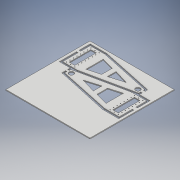
# Autodesk Inventor part: W1support
Saved by Autodesk Inventor 2017 (Build 210142000, 142)
## iProperties
Created: 2016-10-09
Part Number: W1support
Material: Generic
Document SubType Name: Sheet Metal
Designer: aesen
Density: 1 g/cm^3
Sheet Metal Rule: Default_mm
Appearance: Default
Author: aesen
Autodesk Inventor part; units mm, degrees
ref_plane "YZ Plane" through (0, 0, 0) normal (1, 0, 0) x (0, 1, 0)
ref_plane "XZ Plane" through (0, 0, 0) normal (0, 1, 0) x (-1, 0, 0)
ref_plane "XY Plane" through (0, 0, 0) normal (0, 0, 1) x (1, 0, 0)
sketch "Sketch1" plane through (0, 0, 0) normal (0, 0, 1) x (1, 0, 0)
  line L0 (-457.2, 457.2) -> (457.2, 457.2)
  line L1 (457.2, 457.2) -> (457.2, -457.2)
  line L2 (457.2, -457.2) -> (-457.2, -457.2)
  line L3 (-410.8712, 413.3546) -> (-250.8712, 413.3546)
  line L4 (-250.8712, 113.3546) -> (-410.8712, 113.3546)
  line L5 (-410.8712, 113.3546) -> (-410.8712, 413.3546)
  circle A0 centre (-295.7802, 396.0326) radius 3.5
  circle A1 centre (-295.7872, 130.6766) radius 3.7075
  circle A2 centre (-385.5982, 396.0326) radius 3.7075
  circle A3 centre (-340.6821, 395.2343) radius 3.7075
  circle A4 centre (-385.5982, 130.6766) radius 3.5
  circle A5 centre (-340.6892, 129.8783) radius 3.5
  circle A6 centre (-295.7802, 358.1246) radius 3.5
  circle A7 centre (-295.7802, 320.2166) radius 3.5
  circle A8 centre (-295.9938, 282.3086) radius 3.5
  circle A9 centre (-295.7802, 244.4006) radius 3.5
  circle A10 centre (-295.7802, 206.4926) radius 3.5
  circle A11 centre (-295.7802, 168.5846) radius 3.5
  circle A12 centre (-385.5982, 358.1246) radius 3.5
  circle A13 centre (-385.5982, 320.2166) radius 3.5
  circle A14 centre (-385.8118, 282.3086) radius 3.5
  circle A15 centre (-385.5982, 244.4006) radius 3.5
  circle A16 centre (-385.5982, 206.4926) radius 3.5
  circle A17 centre (-385.5982, 168.5846) radius 3.5
  line L6 (-370.8118, 380.2343) -> (-310.9938, 380.2343)
  line L7 (-310.9938, 380.2343) -> (-310.9938, 144.8783)
  line L8 (-310.9938, 144.8783) -> (-370.8118, 144.8783)
  line L9 (-370.8118, 144.8783) -> (-370.8118, 380.2343)
  line L10 (-250.8712, 413.3546) -> (299.1288, 296.4485)
  line L11 (-250.8712, 113.3546) -> (299.1288, 230.2607)
  line L12 (299.1288, 296.4485) -> (299.1288, 230.2607)
  circle A18 centre (258.1288, 263.3546) radius 25.4
  line L13 (-213.1624, 168.8022) -> (-213.1624, 357.9527)
  line L14 (-78.488, 321.6634) -> (-78.488, 205.0454)
  line L15 (-27.0623, 216.039) -> (-27.0622, 310.6699)
  line L16 (-78.488, 321.6634) -> (-213.1624, 357.9527)
  line L17 (-78.488, 205.0454) -> (-213.9712, 168.5846)
  line L18 (-27.0623, 216.039) -> (131.2941, 263.3459)
  line L19 (131.2941, 263.3459) -> (-27.0622, 310.6699)
  line L20 (83.0359, 109.6863) -> (83.0359, -6.9318)
  line L21 (415.4191, -98.6226) -> (415.4191, 201.3774)
  circle A19 centre (390.1461, 32.4235) radius 3.5
  line L22 (375.3597, -67.0988) -> (375.3597, 168.2572)
  line L23 (315.5417, 168.2572) -> (315.5417, -67.0988)
  circle A20 centre (300.3281, 32.4234) radius 3.5
  line L24 (255.4191, -98.6226) -> (415.4191, -98.6226)
  circle A21 centre (390.3597, 70.3315) radius 3.5
  circle A22 centre (300.3281, 108.2394) radius 3.5
  circle A23 centre (390.1461, 108.2395) radius 3.5
  circle A24 centre (390.1461, 146.1474) radius 3.5
  circle A25 centre (300.3281, 146.1474) radius 3.5
  line L25 (375.3597, 168.2572) -> (315.5417, 168.2572)
  line L26 (415.4191, 201.3774) -> (255.4191, 201.3774)
  circle A26 centre (300.5417, 70.3314) radius 3.5
  circle A27 centre (300.3352, -81.3006) radius 3.7075
  circle A28 centre (390.1461, -81.3006) radius 3.5
  circle A29 centre (300.3281, -5.4846) radius 3.5
  circle A30 centre (390.1461, -5.4846) radius 3.5
  circle A31 centre (300.3281, -43.3926) radius 3.5
  circle A32 centre (390.1461, -43.3926) radius 3.5
  line L27 (315.5417, -67.0988) -> (375.3597, -67.0988)
  circle A33 centre (345.2371, -82.0988) radius 3.5
  circle A34 centre (300.3281, 184.0554) radius 3.5
  circle A35 centre (390.1461, 184.0554) radius 3.7075
  circle A36 centre (345.23, 183.2572) radius 3.7075
  line L28 (217.7103, -43.1749) -> (217.7103, 145.9755)
  line L29 (83.0359, 109.6863) -> (217.7103, 145.9755)
  line L30 (83.0359, -6.9318) -> (218.5191, -43.3926)
  line L31 (31.6102, 4.0618) -> (31.6101, 98.6927)
  line L32 (255.4191, -98.6226) -> (-294.5809, 18.2835)
  line L33 (255.4191, 201.3774) -> (-294.5809, 84.4713)
  line L34 (31.6102, 4.0618) -> (-126.7462, 51.3687)
  line L35 (-126.7462, 51.3687) -> (31.6101, 98.6927)
  line L36 (-294.5809, 84.4713) -> (-294.5809, 18.2835)
  circle A37 centre (-253.5809, 51.3774) radius 25.4
  line L37 (-457.2, 457.2) -> (-457.2, -457.2)
  line L38 (-410.6499, 430.1514) -> (-247.3009, 430.1514)
  line L39 (-247.3009, 430.1514) -> (316.104, 310.6699)
  line L40 (316.104, 310.6699) -> (316.104, 220.9277)
  line L41 (316.104, 220.9277) -> (426.288, 220.9277)
  line L42 (426.288, 220.9277) -> (437.7452, 220.9277)
  line L43 (432.0166, 220.9277) -> (432.0166, -119.3062)
  line L44 (432.0166, -119.3062) -> (255.1978, -119.3062)
  line L45 (255.1978, -119.3062) -> (-309.8372, 3.9799)
  line L46 (-309.8372, 3.9799) -> (-309.8372, 95.4348)
  line L47 (-309.8372, 95.4348) -> (-428.7699, 95.4348)
  line L48 (-428.7699, 95.4348) -> (-428.7699, 430.1514)
  line L49 (-428.7699, 430.1514) -> (-410.6499, 430.1514)
  line L50 (299.1288, 282.3086) -> (316.104, 282.3086)
  line L51 (316.104, 253.1545) -> (299.1288, 253.1545)
  line L52 (-428.7699, 310.6699) -> (-410.8712, 310.6699)
  line L53 (-428.7699, 282.3086) -> (-410.8712, 282.3086)
  line L54 (432.0166, 84.4713) -> (415.4191, 84.4713)
  line L55 (432.0166, 43.875) -> (415.4191, 43.875)
  line L56 (-309.8372, 66.8314) -> (-294.5809, 66.8314)
  line L57 (-309.8372, 43.875) -> (-294.5809, 43.875)
  point P0 (0, 0)
  dimension "d3" = 914.4
  dimension "d7" = 300
  dimension "d15" = 17.322
  dimension "d16" = 17.322
  dimension "d19" = 44.909
  dimension "d25" = 44.909
  dimension "d62" = 235.356
  dimension "d63" = 59.818
  dimension "d64" = 15
  dimension "d65" = 15
  dimension "d66" = 15
  dimension "d67" = 15
  dimension "d75" = 550
  dimension "d76" = 550
  dimension "d102" = 914.4
  dimension "d103" = 16.7968
  constraints: 116 end point, 38 centre point, 21 point on line, 10 perpendicular, 8 horizontal, 7 parallel, 3 vertical, 1 midpoint
  measures "d3" distance between parallel lines of L2 L0
  measures "d7" distance between parallel lines of L4 L3
  measures "d15" distance from line of L4 A1.centre
  measures "d16" distance from line of L3 A0.centre
  measures "d19" distance of A0.centre A3.centre
  measures "d25" distance of A5.centre A1.centre
  measures "d62" distance between parallel lines of L8 L6
  measures "d63" distance between parallel lines of L9 L7
  measures "d64" distance from line of L6 A3.centre
  measures "d65" distance from line of L8 A5.centre
  measures "d66" distance from line of L7 A8.centre
  measures "d67" distance from line of L9 A14.centre
  measures "d75" horizontal distance of L3.end L10.end
  measures "d76" horizontal distance of L4.start L11.end
  measures "d102" distance of L0.start L0.end
  measures "d103" distance between parallel lines of L38 L3
extrude "Extrusion5" add sketch "Sketch1" along normal blind 9.525 contours L0 L1 L2 L37 | L3 L10 L12 L11 L4 L5 | L5 L53 L48 L52 | L50 L40 L51 L12 | L56 L36 L57 L46 | L36 L33 L26 L21 L24 L32 | L43 L55 L21 L54
equation "\"BendRadius\" = Thickness"
equation "\"BendReliefWidth\" = Thickness"
equation "\"BendReliefDepth\" = 0.5 * Thickness"
equation "\"CornerReliefSize\" = 4 * Thickness"
equation "\"MinimumRemnant\" = 2 * Thickness"
equation "\"TransitionRadius\" = BendRadius"
equation "\"JacobiRadiusSize\" = BendRadius"
equation "\"GapSize\" = Thickness"
equation "\"Thickness\" = 0.5"
body "Solid5"
